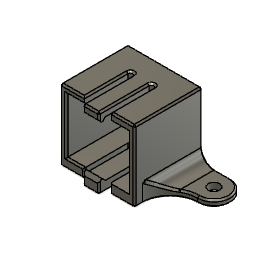
wago (Autodesk Fusion 360 design; units mm, degrees)
Autodesk Fusion 360 part; units mm, degrees
sketch "Sketch1" plane through (0, 0, 0) normal (0, 1, 0) x (1, 0, 0)
  line L0 (0, 19) -> (19, 19)
  line L1 (19, 19) -> (19, 0)
  line L2 (19, 0) -> (0, 0)
  line L3 (0, 0) -> (0, 19)
  line L4 (-2, 21) -> (19, 21)
  line L5 (19, 21) -> (19, -2)
  line L6 (19, -2) -> (-2, -2)
  line L7 (-2, -2) -> (-2, 21)
  circle A0 centre (3, 29.5) radius 1.75
  line L8 (8, 29.5) -> (8, 21)
  line L9 (-2, 29.5) -> (-2, 21)
  arc A1 (8, 29.5) -> (-2, 29.5) centre (3, 29.5) ccw
  line L10 (19, 4.5) -> (19, 12.5)
  line L11 (0, 9.5) -> (19, 9.5)
  line L12 (19, 13.5) -> (5.5, 13.5)
  line L13 (5.5, 5.5) -> (19, 5.5)
  line L14 (19, 5.5) -> (19, 13.5)
  line L15 (5.5, 12) -> (19, 12)
  line L16 (5.5, 7) -> (19, 7)
  arc A2 (5.5, 13.5) -> (5.5, 12) centre (5.5, 12.75) ccw
  arc A3 (5.5, 7) -> (5.505, 5.5) centre (5.5, 6.25) ccw
  line L17 (19, 12) -> (21, 12)
  line L18 (21, 12) -> (21, 7)
  line L19 (21, 7) -> (19, 7)
  arc A4 (-2, -10.5) -> (8, -10.5) centre (3, -10.5) ccw
  circle A5 centre (3, -10.5) radius 1.75
  line L20 (-2, -10.5) -> (-2, -2)
  line L21 (8, -10.5) -> (8, -2)
  dimension "d1" = 19
  dimension "d2" = 19
  dimension "d3" = 21
  dimension "d4" = 23
  dimension "d6" = 2
  dimension "d13" = 10
  dimension "d26" = 2
  dimension "d27" = 3.5
  dimension "d31" = 1.5
  dimension "d32" = 2
  dimension "d33" = 5
  dimension "d34" = 13.5
  dimension "d35" = 13.5
  dimension "d56" = 40
  constraint horizontal L0
  constraint vertical L1
  constraint horizontal L2
  constraint vertical L3
  constraint horizontal L4
  constraint vertical L5
  constraint horizontal L6
  constraint vertical L7
  constraint coincident L2.end L3.start
  constraint concentric A0 A1
  constraint coincident L4 L8.end
  constraint tangent L8 A1
  constraint perpendicular L4 L8
  constraint coincident L4 L7.end
  constraint tangent L9 A1
  constraint perpendicular L4 L9
  constraint vertical L10
  constraint coincident L1 L10.end
  constraint coincident L3 L11.start
  constraint coincident L1 L11.end
  constraint horizontal L11
  constraint horizontal L12
  constraint horizontal L13
  constraint vertical L14
  constraint coincident L5 L12.start
  constraint symmetric L11 L12 L13
  constraint coincident L14 L15.end
  constraint coincident L14 L16.end
  constraint parallel L13 L16
  constraint symmetric L11 L15.end L16.end
  constraint parallel L12 L15
  constraint tangent L15 A2
  constraint tangent L12 A2
  constraint tangent L16 A3
  constraint tangent L13 A3
  constraint coincident A3 L13.start
  constraint perpendicular L1 L17
  constraint perpendicular L17 L18
  constraint horizontal L19
  constraint coincident L4.start L7.end
  constraint symmetric L0 L2 L11
  constraint symmetric A0 L11 A5
  constraint symmetric L8.start L11 A4.end
  constraint symmetric L8.end L11 L21.end
  constraint symmetric L9.start L11 A4.start
  constraint symmetric L4.start L11 L6.end
  constraint symmetric A1 L11 A4
  measures "d1" distance of L0.start L0.end
  measures "d2" distance of L0.start L2.end
  measures "d3" distance of L4.start L4.end
  measures "d4" distance of L4.start L6.end
  measures "d6" horizontal distance of L2.end L6.end
  measures "d13" diameter of A1
  measures "d26" vertical distance of L2.end L6.end
  measures "d27" diameter of A0
  measures "d31" distance of L12.start L15.end
  measures "d32" distance of L16.end L18.end
  measures "d33" distance of L17.end L18.end
  measures "d34" distance of L16.end L16.start
  measures "d35" distance of L15.end L15.start
  measures "d56" distance of A0.centre A4.centre
extrude "Extrude1" add sketch "Sketch1" along normal blind 22 contours L0 L2 L3 L4 L5 L6 L7 | L0 L1 L3 L5 L10 L11 L12 L14 L15 A2 | L1 L2 L3 L5 L10 L11 L13 L14 L16 A3 | L1 L5 L10 L12 L14 L15 A2 | L1 L5 L10 L13 L14 L16 A3
extrude "Extrude2" cut sketch "Sketch1" along normal blind 17 from surface at 3 contours L0 L1 L3 L5 L10 L11 L12 L14 L15 A2 | L1 L2 L3 L5 L10 L11 L13 L14 L16 A3 | L1 L5 L10 L12 L14 L15 A2 | L1 L5 L10 L13 L14 L16 A3
extrude "Extrude3" add sketch "Sketch1" along normal blind 2 contours L0 L1 L3 L5 L10 L11 L12 L14 L15 A2 | L1 L2 L3 L5 L10 L11 L13 L14 L16 A3 | L1 L5 L10 L12 L14 L15 A2 | L4 L8 L9 A1 | L1 L5 L10 L13 L14 L16 A3 | L6 A4 L20 L21
extrude "Extrude4" cut sketch "Sketch1" along normal through all contours L1 L5 L10 L12 L14 L15 A2 | L1 L5 L10 L13 L14 L16 A3
extrude "Extrude5" add sketch "Sketch1" along normal blind 3 from surface at 19 contours L1 L5 L10 L14 L17 L18 L19
extrude "Extrude6" add sketch "Sketch1" along normal blind 4 contours L1 L5 L10 L14 L17 L18 L19
chamfer "Chamfer1" distance 1 angle 45 4 edges at (19, 19, -9.5) (21, 19, -9.5) (19, 4, -9.5) (21, 4, -9.5)
fillet "Fillet1" radius 8.5 2 edges at (8, 1, -21) (8, 1, 2)
fillet "Fillet2" radius 4 2 edges at (7.25, 2, -21) (7.25, 2, 2)
chamfer "Chamfer4" distance 0.5 angle 45 49 edges at (8.5, 22, 2) (8.5, 22, -21) (17.75, 0, -21) (10.4896, 0, -23.4896) (3, 0, -34.5) (-2, 0, -9.5) (3, 0, 15.5) (10.4896, 0, 4.4896) (17.75, 0, 2) (19, 22, -1.75) (19, 20, -2.75) (19, 11.5, 0) (19, 11.5, -19) (19, 21, -13.5) (19, 1.5, -13.5) (21, 1.5, -12) (19, 1.5, -5.5) (19, 3, -2.75) (21, 22, -9.5) (21, 21, -12) (21, 21, -7) (12.25, 22, -5.5) (4.75, 22, -6.25) (13.25, 22, -7) (13.25, 22, -12) (4.75, 22, -12.75) (12.25, 22, -13.5) (-2, 22, -9.5) (19, 11, -21) (-2, 12, -21) (3, 2, -34.5) (8.3282, 2, -27.1594) (-2, 2, -25.25) (19, 11, 2) (19, 0, -1.75) (19, 0, -17.25) (21, 0, -9.5) (21, 1.5, -7) (13.25, 0, -7) (4.75, 0, -6.25) (12.25, 0, -5.5) (13.25, 0, -12) (4.75, 0, -12.75) (12.25, 0, -13.5) (19, 22, -17.25) (-2, 12, 2) (-2, 2, 6.25) (3, 2, 15.5) (8.3282, 2, 8.1594)
move_body "Move1" bodies 1 to x (0, 0, 1) y (0, 1, 0) z (-1, 0, 0) at (0, 0, 0)
